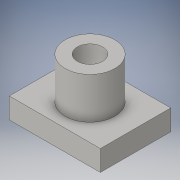
# Autodesk Inventor part: imusupport
Saved by Autodesk Inventor 2016 (Build 200138000, 138)
## iProperties
Created: 2017-04-12
Part Number: imusupport
Material: Generic
Document SubType Name: Modeling
Designer: Evan Phil George
Density: 1 g/cm^3
Appearance: Default
Author: Evan Phil George
## iProperties of the stored document imusupport_3DPrint.ipt
Created: 2017-04-12
Part Number: imusupport_3DPrint
Material: Generic
Document SubType Name: Modeling
Designer: Evan Phil George
Density: 1 g/cm^3
Appearance: Default
Author: Evan Phil George
Autodesk Inventor part; units mm, degrees
ref_plane "YZ Plane" through (0, 0, 0) normal (1, 0, 0) x (0, 1, 0)
ref_plane "XZ Plane" through (0, 0, 0) normal (0, 1, 0) x (-1, 0, 0)
ref_plane "XY Plane" through (0, 0, 0) normal (0, 0, 1) x (1, 0, 0)
sketch "Sketch1" plane through (0, 0, 0) normal (0, 1, 0) x (-1, 0, 0)
  line L0 (11, -8.5) -> (-11, -8.5)
  line L1 (-11, -8.5) -> (-11, 8.5)
  line L2 (-11, 8.5) -> (11, 8.5)
  line L3 (11, 8.5) -> (11, -8.5)
  line L4 (11, -8.5) -> (-11, 8.5) construction
  line L5 (-11, -8.5) -> (11, 8.5) construction
  point P0 (0, 0)
  dimension "d0" = 22
  dimension "d1" = 17
  constraints: 12 end point, 2 midpoint, 2 parallel, 1 horizontal, 1 perpendicular
  measures "d0" distance of L1.end L2.end
  measures "d1" distance of L0.end L1.end
extrude "Extrusion1" add sketch "Sketch1" along normal blind 5
sketch "Sketch2" plane through (0, 5, 0) normal (0, 1, 0) x (1, 0, 0)
  circle A0 centre (0, 0) radius 6
  circle A1 centre (0, 0) radius 3.05
  dimension "d4" = 12
  dimension "d5" = 6.1
  constraints: 2 centre point, 2 coincident
  measures "d4" diameter of A0
  measures "d5" diameter of A1
extrude "Extrusion2" add sketch "Sketch2" along normal blind 10
body "Solid1"
